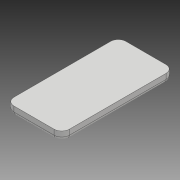
# Autodesk Inventor part: basic shape
Saved by Autodesk Inventor 2017 (Build 210142000, 142)
## iProperties
Created: 2016-05-26
Part Number: basic shape
Material: Generic
Document SubType Name: Modeling
Designer: ari
Density: 1 g/cm^3
Appearance: Default
Author: ari
Autodesk Inventor part; units mm, degrees
ref_plane "YZ Plane" through (0, 0, 0) normal (1, 0, 0) x (0, 1, 0)
ref_plane "XZ Plane" through (0, 0, 0) normal (0, 1, 0) x (-1, 0, 0)
ref_plane "XY Plane" through (0, 0, 0) normal (0, 0, 1) x (1, 0, 0)
sketch "Sketch1" plane through (0, 0, 0) normal (0, 0, 1) x (1, 0, 0)
  line L0 (-32.5, -65.6) -> (32.5, -65.6)
  line L1 (32.5, -65.6) -> (32.5, 65.6)
  line L2 (32.5, 65.6) -> (-32.5, 65.6)
  line L3 (-32.5, 65.6) -> (-32.5, -65.6)
  line L4 (-32.5, -65.6) -> (32.5, 65.6) construction
  line L5 (32.5, -65.6) -> (-32.5, 65.6) construction
  point P0 (0, 0)
  dimension "d0" = 65
  dimension "d1" = 131.2
  constraints: 12 end point, 2 midpoint, 2 parallel, 1 horizontal, 1 perpendicular
  measures "d0" distance of L1.end L2.end
  measures "d1" distance of L0.end L1.end
extrude "Extrusion1" add sketch "Sketch1" along normal blind 9.6
fillet "Fillet1" radius 3.5 4 edges at (32.5, 0, 0) (0, 65.6, 0) (-32.5, 0, 0) (0, -65.6, 0)
fillet "Fillet1" radius 9 4 edges at (32.5, 65.6, 4.8) (-32.5, 65.6, 4.8) (-32.5, -65.6, 4.8) (32.5, -65.6, 4.8)
body "Solid1"
